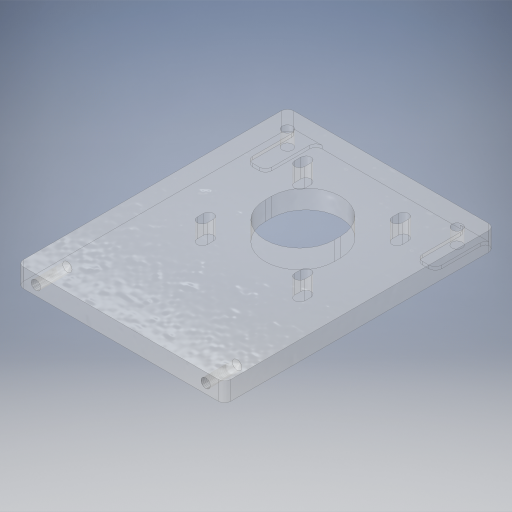
# Autodesk Inventor part: getriebe_halterung
Saved by Autodesk Inventor 2023 (Build 270158000, 158)
## iProperties
Company: HTBLA Kaindorf
RuleStatus: InUse
Created: 2023-01-09
Part Number: getriebe_halterung
Project: Zeichenmaschine
Material: Acryl
Description: Zeichenmaschine_stepper_getriebe_halterung
Document SubType Name: Modeling
Designer: goteln20
Density: 1.188 g/cm^3
Appearance: Transparent - farblos
Mass: 36.4953 g
Surface Area: 132.786 cm^2
Volume: 30.72 cm^3
AfterDocNew0: iProperties-Editor_aufrufen
Author: eligo
Keywords: 23
Autodesk Inventor part; units mm, degrees
ref_plane "YZ Plane" through (0, 0, 0) normal (1, 0, 0) x (0, 1, 0)
sketch "Skizze3" plane through (0, 0, 0) normal (0, 0, 1) x (1, 0, 0)
  line L0 (0, 0) -> (-86, 0)
  line L1 (-86, 0) -> (-86, -66)
  line L2 (-86, -66) -> (0, -66)
  line L3 (0, -66) -> (0, 0)
  line L4 (-57.9, -33) -> (-86, -33) construction
  line L5 (-42.4, -48.5) -> (-73.4, -48.5) construction
  line L6 (-74.4, -48.5) -> (-72.4, -48.5) construction
  line L7 (-74.4, -46.9) -> (-72.4, -46.9)
  line L8 (-72.4, -50.1) -> (-74.4, -50.1)
  arc A0 (-74.4, -46.9) -> (-74.4, -50.1) centre (-74.4, -48.5) ccw
  arc A1 (-72.4, -50.1) -> (-72.4, -46.9) centre (-72.4, -48.5) ccw
  line L9 (-43.4, -48.5) -> (-41.4, -48.5) construction
  line L10 (-43.4, -50.1) -> (-41.4, -50.1)
  line L11 (-41.4, -46.9) -> (-43.4, -46.9)
  arc A2 (-43.4, -46.9) -> (-43.4, -50.1) centre (-43.4, -48.5) ccw
  arc A3 (-41.4, -50.1) -> (-41.4, -46.9) centre (-41.4, -48.5) ccw
  line L12 (-74.4, -19.1) -> (-72.4, -19.1)
  line L13 (-72.4, -15.9) -> (-74.4, -15.9)
  arc A4 (-74.4, -15.9) -> (-74.4, -19.1) centre (-74.4, -17.5) ccw
  arc A5 (-72.4, -19.1) -> (-72.4, -15.9) centre (-72.4, -17.5) ccw
  line L14 (-43.4, -15.9) -> (-41.4, -15.9)
  line L15 (-41.4, -19.1) -> (-43.4, -19.1)
  arc A6 (-43.4, -15.9) -> (-43.4, -19.1) centre (-43.4, -17.5) ccw
  arc A7 (-41.4, -19.1) -> (-41.4, -15.9) centre (-41.4, -17.5) ccw
  line L16 (-58.9, -33) -> (-56.9, -33) construction
  line L17 (-58.9, -44) -> (-56.9, -44)
  line L18 (-56.9, -22) -> (-58.9, -22)
  arc A8 (-58.9, -22) -> (-58.9, -44) centre (-58.9, -33) ccw
  arc A9 (-56.9, -44) -> (-56.9, -22) centre (-56.9, -33) ccw
  point P0 (-57.9, -48.5)
  dimension "d4" = 86
  dimension "d5" = 66
  dimension "d44" = 31
  dimension "d53" = 28.1
  dimension "d54" = 15.5
  dimension "d55" = 1.6
  dimension "d56" = 2
  dimension "d57" = 1.6
  dimension "d58" = 2
  dimension "d59" = 2
  dimension "d60" = 11
  constraints: 44 end point, 20 point on circle, 12 symmetric about line, 12 tangent, 10 centre point, 5 horizontal, 5 midpoint, 5 parallel, 2 horizontal alignment, 1 perpendicular, 1 point on line, 1 vertical alignment, 4 other
  measures "d4" distance of L1.end L2.end
  measures "d5" distance of L0.end L1.end
  measures "d44" distance of L5.end L5.start
  measures "d53" distance from line of L1 L4.start
  measures "d54" horizontal distance of L5.end L4.start
  measures "d55" radius of A1
  measures "d56" distance of L8.start L8.end
  measures "d57" radius of A3
  measures "d58" distance of L11.start L11.end
  measures "d59" distance of L18.start L18.end
  measures "d60" radius of A9
extrude "Extrusion3" add sketch "Skizze3" along normal blind 6 contours L3 L2 L1 L0 | L7 A1 L8 A0 | A2 L11 A3 L10 | A4 L13 A5 L12 | L14 A7 L15 A6 | A8 L18 A9 L17
sketch "Skizze4" plane through (0, -66, 0) normal (1, 0, 0) x (0, 0, -1)
  line L0 (0, 0) -> (-6, 0) projected
  line L1 (-3, 0) -> (-3, 70) construction
  line L2 (0, 66) -> (0, 0) projected
  line L3 (0, 66) -> (-6, 66) projected
  point P0 (-3, 60)
  point P1 (-3, 6)
  dimension "d10" = 6
  dimension "d11" = 6
  constraints: 2 end point, 2 point on line, 1 midpoint, 1 parallel, 1 other
  measures "d11" distance from line of L0 point (-3, 6)
hole "Bohrung1" at (0, -6, 3) at (0, -60, 3) direction (-1, 0, 0) diameter 3 depth 10 tip angle 118
thread "Gewinde2" size "M3x0.5" class "6H" standard "ISO Metric profile" length 8
thread "Gewinde3" size "M3x0.5" class "6H" standard "ISO Metric profile" length 8
sketch "Skizze5" plane through (0, 0, 6) normal (0, 0, 1) x (1, 0, 0)
  line L0 (0, -60) -> (-86, -60) construction
  line L1 (-86, 0) -> (-86, -66) projected
  line L2 (-70, -63.025) -> (-86, -63.025)
  line L3 (-86, -63.025) -> (-86, -56.975)
  line L4 (-86, -56.975) -> (-70, -56.975)
  line L5 (-70, -56.975) -> (-70, -63.025)
  line L6 (0, -66) -> (0, 0) projected
  line L7 (0, -33) -> (-86, -33) construction
  line L8 (-70, -2.975) -> (-86, -2.975)
  line L9 (-86, -2.975) -> (-86, -9.025)
  line L10 (-86, -9.025) -> (-70, -9.025)
  line L11 (-70, -9.025) -> (-70, -2.975)
  point P0 (0, -6)
  point P1 (-80, -60)
  point P2 (-70, -60)
  point P3 (-80, -6)
  point P4 (-86, -2.975)
  point P5 (-86, -9.025)
  dimension "d26" = 6
  dimension "d34" = 16
  dimension "d35" = 6.05
  constraints: 20 end point, 5 symmetric about line, 4 point on line, 3 horizontal, 3 midpoint, 2 parallel, 1 perpendicular
  measures "d26" distance from line of L1 point (-80, -60)
  measures "d34" distance of L2.start L2.end
  measures "d35" distance of L4.end L2.start
hole "Bohrung2" at (-80, -60, 6) at (-80, -6, 6) direction (0, 0, -1) diameter 3.3 depth 8.1
sketch "Skizze6" plane through (0, 0, 0) normal (0, 0, -1) x (-1, 0, 0)
  line L0 (86, -9.025) -> (70, -9.025) projected
  line L1 (70, -9.025) -> (70, -2.975) projected
  line L2 (70, -2.975) -> (86, -2.975) projected
  line L3 (86, -56.975) -> (70, -56.975) projected
  line L4 (70, -63.025) -> (86, -63.025) projected
  line L5 (70, -56.975) -> (70, -63.025) projected
  line L6 (86, 0) -> (86, -66) projected
  point P0 (0, 0)
  point P1 (80, -6)
extrude "Extrusion5" cut sketch "Skizze6" against normal blind 1
fillet "Rundung3" radius 2 4 edges at (0, -66, 3) (0, 0, 3) (-86, -66, 3) (-86, 0, 3)
fillet "Rundung4" radius 2 8 edges at (-86, -2.975, 0.5) (-86, -9.025, 0.5) (-70, -2.975, 0.5) (-70, -9.025, 0.5) (-86, -56.975, 0.5) (-86, -63.025, 0.5) (-70, -56.975, 0.5) (-70, -63.025, 0.5)
extrude "Extrusion6" cut sketch "Skizze3" along normal blind 10 contours L7 A1 L8 A0 | A2 L11 A3 L10 | A4 L13 A5 L12 | L14 A7 L15 A6 | A8 L18 A9 L17
ref_plane "Arbeitsebene1" through (-73.4, -48.5, 0) normal (-1, 0, 0) x (0, 0, 1)
ref_plane "Arbeitsebene2" through (-42.4, -48.5, 0) normal (-1, 0, 0) x (0, 0, 1)
equation "\"d54\" = 0.5 * d44"
equation "\"d57\" = d55"
